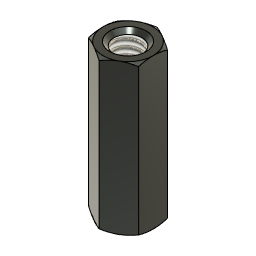
OH2A7A1-100 - AIRSPEED INDICATOR (Autodesk Fusion 360 archive; units mm, degrees)
design "91780A028 - STANDOFF, #2-56 X .375, .125 HEX, FEMALE, 6061"
description: STANDOFF, #2-56 X .375, .125 HEX, FEMALE, 6061
part number: 91780A028
Autodesk Fusion 360 part; units mm, degrees
note: some values were not read from the file. Chosen so that the rebuilt part matches the saved one: how an offset face is resized.
sketch "Sketch1" plane through (0, 0, 0) normal (0, 0, 1) x (1, 0, 0)
  line L0 (1.5875, 0.9165) -> (0, 1.8331)
  line L1 (0, 1.8331) -> (-1.5875, 0.9165)
  line L2 (-1.5875, 0.9165) -> (-1.5875, -0.9165)
  line L3 (-1.5875, -0.9165) -> (0, -1.8331)
  line L4 (0, -1.8331) -> (1.5875, -0.9165)
  line L5 (1.5875, -0.9165) -> (1.5875, 0.9165)
  circle A0 centre (0, 0) radius 1.5875 construction
  dimension "d4" = 3.175
  constraint coincident A0.centre origin
  constraint vertical L5
  constraint tangent L0 A0
  measures "d4" distance of L2 L5
extrude "Extrude1" add sketch "Sketch1" along normal mid plane 9.525
sketch "Sketch2" plane through (0, 0, 0) normal (1, 0, 0) x (0, 1, 0)
  line L0 (1.8331, 4.7625) -> (-1.8331, 4.7625)
  line L1 (-1.8331, -4.7625) -> (1.8331, -4.7625)
  line L2 (-1.5875, 0) -> (-1.5875, 4.7625) construction
  line L3 (-1.5875, 0) -> (-1.5875, -4.7625) construction
  line L4 (-1.8331, 4.7625) -> (-1.8331, 4.6207)
  line L5 (-1.8331, 4.6207) -> (-1.5875, 4.7625)
  line L6 (-1.5875, 0) -> (0, 0) construction
  line L7 (0, 0) -> (0, 4.7625)
  line L8 (-1.8331, -4.6207) -> (-1.5875, -4.7625)
  line L9 (-1.8331, -4.7625) -> (-1.8331, -4.6207)
  point P0 (-1.5875, 0)
  point P1 (1.5875, 0)
  dimension "d7" = 30
  constraint coincident P0 L2.start
  constraint coincident L0 L2.end
  constraint perpendicular L0 L2
  constraint coincident L1 L3.end
  constraint perpendicular L1 L3
  constraint coincident L0.end L4.start
  constraint perpendicular L0 L4
  constraint coincident L6.end L7.start
  constraint midpoint L0 L7.end
  constraint symmetric L2.end L6 L3.end
  constraint symmetric L0.end L6 L1.start
  constraint symmetric L4.end L6 L8.start
  measures "d7" angle of L0 L5
revolve "Revolve1" cut sketch "Sketch2" angle 360 about axis through (0, 0, 0) along (0, 0, 1)
sketch "Sketch3" plane through (0, 0, 0) normal (0, 1, 0) x (1, 0, 0)
  line L0 (-1.5875, -4.7625) -> (1.5875, -4.7625)
  line L1 (1.5875, 4.7625) -> (-1.5875, 4.7625)
  line L2 (0, -4.7625) -> (0, 4.7625)
  line L3 (0, -4.1891) -> (0.5734, -4.1891)
  line L4 (0.5734, -4.1891) -> (1.1468, -4.7625)
  line L5 (0, 0) -> (1.5875, 0) construction
  line L6 (0, 4.1891) -> (0.5734, 4.1891)
  line L7 (0.5734, 4.1891) -> (1.1468, 4.7625)
  dimension "d9" = 45
  dimension "d10" = 2.2936
  dimension "d11" = 1.1468
  constraint midpoint L0 L2.start
  constraint midpoint L1 L2.end
  constraint coincident L2 L3.start
  constraint perpendicular L2 L3
  constraint coincident L0 L4.end
  constraint coincident L5.start origin
  constraint perpendicular L2 L5
  constraint vertical L0.end L5.end
  constraint symmetric L3.start L5 L6.start
  constraint symmetric L3.end L5 L6.end
  constraint symmetric L4.end L5 L7.end
  measures "d9" angle of L0 L4
sketch "Sketch4" plane through (0, 0, 4.7625) normal (0, 0, 1) x (-1, 0, 0)
  arc A0 (-0.7937, -1.3748) -> (0.7937, -1.3748) centre (0, 0) ccw
  arc A1 (0.7937, -1.3748) -> (1.5875, 0) centre (0, 0) ccw
  arc A2 (1.5875, 0) -> (0.7937, 1.3748) centre (0, 0) ccw
  arc A3 (0.7937, 1.3748) -> (-0.7937, 1.3748) centre (0, 0) ccw
  arc A4 (-0.7937, 1.3748) -> (-1.5875, 0) centre (0, 0) ccw
  arc A5 (-1.5875, 0) -> (-0.7937, -1.3748) centre (0, 0) ccw
  constraint coincident A0.centre A1.centre
hole "Hole1" at (0, 0, 4.7625) direction (0, 0, -1) diameter 1.778 end through all
thread "Thread1" "ANSI Unified Screw Threads 0.086(#2) 2-56 UNC 2B" major diameter 2.1844 minor diameter 1.7831 pitch 0.4536 angle 60 resizes the face on face at (0.0715, -0.8861, 1.5875)
revolve "Revolve2" cut sketch "Sketch3" angle 360 about axis through (0, 0, 4.7625) along (0, 0, -1)
equation "Length = ( 3 / 8 ) * 1 in" comment "Standoff length"
equation "HexWidth = ( 1 / 8 ) * 1 in" comment "Hex Size (opposite sides)"
equation "MajorDia = 0.086 in" comment "Thread nominal major diameter"
equation "d4 = HexWidth"
equation "d5 = Length"
equation "d10 = MajorDia * 1.05"
equation "d11 = d10 / 2"
